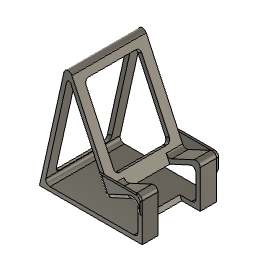
MultimeterStand (Autodesk Fusion 360 design; units mm, degrees)
Autodesk Fusion 360 part; units mm, degrees
sketch "Sketch11" plane through (0, 0, 0) normal (0, 1, 0) x (1, 0, 0)
  line L0 (0, 0) -> (0, -35) construction
  line L1 (0, -35) -> (38.064927, -52.749967)
  line L2 (0, -35) -> (42, -35) construction
  line L3 (38.064927, -52.749967) -> (38.064927, 0)
  line L4 (0, -35) -> (-48.072827, -138.092511)
  line L5 (0, -35) -> (131.25, -35) construction
  line L6 (-48.072827, -138.092511) -> (-53.072827, -138.092511)
  line L7 (0, 0) -> (61.000001, 0) construction
  line L8 (-53.072827, -138.092511) -> (-83.6872, 0)
  line L9 (-53.072827, -138.092511) -> (72.884225, -138.092511) construction
  line L10 (0, 0) -> (-120, 0) construction
  line L11 (-83.6872, 0) -> (38.064927, 0)
  dimension "d68" = 35
  dimension "d69" = 42
  dimension "d70" = 25
  dimension "d71" = 115
  dimension "d72" = 113.75
  dimension "d73" = 5
  dimension "d81" = 102.5
  constraint vertical L0
  constraint coincident L0.start L7.start
  constraint horizontal L2
  constraint vertical L3
  constraint horizontal L5
  constraint horizontal L6
  constraint perpendicular L0 L7
  constraint horizontal L9
  constraint horizontal L10
  constraint coincident L8.end L10
  measures "d68" distance of L0.start L0.end
  measures "d70" angle of L1 L2
  measures "d71" angle of L4 L5
  measures "d81" angle of L8 L9
extrude "Extrude16" add sketch "Sketch11" along normal blind 88 contours L1 L3 L4 L6 L8 L11 picked at (-45.586676, -57.697504) makes body 1
sketch "Sketch12" plane through (38.064927, 0, 0) normal (1, 0, 0) x (0, 1, 0)
  line L0 (0, 52.749967) -> (0, 0)
  line L1 (88, 0) -> (88, 52.749967)
  line L2 (88, 52.749967) -> (0, 52.749967)
  line L3 (44, 52.749967) -> (43.238153, 0) construction
  line L4 (68.619076, 52.749967) -> (18.619076, 52.749967)
  line L5 (18.619076, 52.749967) -> (18.619076, 0)
  line L6 (18.619076, 0) -> (68.619076, 0)
  line L7 (68.619076, 0) -> (68.619076, 52.749967)
  line L8 (68.619076, 52.749967) -> (18.619076, 0) construction
  line L9 (18.619076, 52.749967) -> (68.619076, 0) construction
  line L10 (0, 0) -> (88, 0)
  point P0 (43.619076, 26.374983)
  dimension "d77" = 50
  constraint horizontal L4
  constraint perpendicular L4 L5
  constraint parallel L4 L6
  constraint parallel L5 L7
  constraint collinear L2 L4
extrude "Extrude17" cut sketch "Sketch12" along normal up to surface contours L2 L4 L5 L6 L7 L10 picked at (51.95241, 17.583322) end surface through (0, 0, 35) normal (0.90630779, 0, 0.42261826) offset 0 bodies 1
sketch "Sketch13" plane through (0, 0, 0) normal (0, -1, 0) x (1, 0, 0)
  line L0 (38.064927, 52.749967) -> (0, 35)
  line L1 (0, 35) -> (-48.072827, 138.092511)
  line L2 (-48.072827, 138.092511) -> (-53.072827, 138.092511)
  line L3 (-53.072827, 138.092511) -> (-83.6872, 0)
  line L4 (-83.6872, 0) -> (38.064927, 0)
  line L5 (38.064927, 0) -> (38.064927, 52.749967)
  line L6 (33.064927, 5) -> (33.064927, 44.901539)
  line L7 (33.064927, 44.901539) -> (-2.418448, 28.35537)
  line L8 (-2.418448, 28.35537) -> (-49.768252, 129.897354)
  line L9 (-49.768252, 129.897354) -> (-77.457329, 5)
  line L10 (-77.457329, 5) -> (33.064927, 5)
extrude "Extrude18" cut sketch "Sketch13" against normal up to surface (88 mm away) contours L6 L7 L8 L9 L10 picked at (-43.214676, 54.417574) bodies 1
sketch "Sketch14" plane through (13.405778, 0, 6.251217) normal (0.906308, 0, 0.422618) x (0, 1, 0)
  line L0 (18.619076, 30.468461) -> (68.619076, 30.468461) construction
  line L1 (68.619076, 30.468461) -> (68.619076, 35) construction
  line L2 (68.619076, 35) -> (88, 35) construction
  line L3 (88, 35) -> (88, 138.092511) construction
  line L4 (88, 138.092511) -> (0, 138.092511) construction
  line L5 (0, 138.092511) -> (0, 35) construction
  line L6 (0, 35) -> (18.619076, 35) construction
  line L7 (18.619076, 35) -> (18.619076, 30.468461) construction
  line L8 (0, 138.092511) -> (88, 35) construction
  line L9 (72, 130.296255) -> (16, 130.296255)
  line L10 (11, 125.296255) -> (11, 47.796255)
  line L11 (16, 42.796255) -> (72, 42.796255)
  line L12 (77, 47.796255) -> (77, 125.296255)
  line L13 (77, 130.296255) -> (11, 42.796255) construction
  line L14 (11, 130.296255) -> (77, 42.796255) construction
  line L15 (18.619076, 26.720773) -> (68.619076, 26.720773)
  line L16 (68.619076, 26.720773) -> (68.619076, 31.720773)
  line L17 (68.619076, 31.720773) -> (88, 31.720773)
  line L18 (88, 31.720773) -> (88, 145.470773)
  line L19 (88, 145.470773) -> (0, 145.470773)
  line L20 (0, 145.470773) -> (0, 31.720773)
  line L21 (0, 31.720773) -> (18.619076, 31.720773)
  line L22 (18.619076, 31.720773) -> (18.619076, 26.720773)
  arc A0 (16, 130.296255) -> (11, 125.296255) centre (16, 125.296255) ccw
  arc A1 (77, 125.296255) -> (72, 130.296255) centre (72, 125.296255) ccw
  arc A2 (72, 42.796255) -> (77, 47.796255) centre (72, 47.796255) ccw
  arc A3 (11, 47.796255) -> (16, 42.796255) centre (16, 47.796255) ccw
  point P0 (44, 86.546255)
  dimension "d101" = 66
  dimension "d102" = 87.5
  dimension "d105" = 5
  constraint coincident L2.end L3.start
  constraint horizontal L9
  constraint perpendicular L9 L10
  constraint parallel L9 L11
  constraint parallel L10 L12
  constraint tangent L10 A0
  constraint tangent L9 A0
  constraint tangent L9 A1
  constraint tangent L12 A1
  constraint equal A0 A1
  constraint tangent L12 A2
  constraint tangent L11 A2
  constraint equal A0 A2
  constraint tangent L11 A3
  constraint tangent L10 A3
  constraint equal A0 A3
  measures "d105" radius of A0
fillet "Fillet5" radius 5 6 edges at (38.064927, 78.309538, 52.749967) (38.064927, 9.309538, 52.749967) (0, 9.309538, 35) (0, 78.309538, 35) (-48.072827, 44, 138.092511) (-53.072827, 44, 138.092511) on bodies 1
fillet "Fillet6" radius 2.5 1 edges at (-49.768252, 44, 129.897354) on bodies 1
fillet "Fillet6" radius 5 6 edges at (-77.457329, 44, 5) (33.064927, 9.309538, 5) (33.064927, 78.309538, 5) (33.064927, 78.309538, 44.901539) (33.064927, 9.309538, 44.901539) (-2.418448, 44, 28.35537) on bodies 1
extrude "Extrude19" cut sketch "Sketch14" along normal up to surface contours L9 L10 L11 L12 A0 A1 A2 A3 picked at (33, 99.462922) end surface through (-53.072827, 0, 138.092511) normal (-0.97629601, 0, 0.21643961) offset 0 bodies 1
sketch "Sketch15" plane through (0, 0, 0) normal (0, -1, 0) x (1, 0, 0)
  arc A0 (-4.531539, 32.886909) -> (2.113091, 30.468461) centre (0, 35) ccw
  line L0 (2.113091, 30.468461) -> (25.951836, 41.58465)
  arc A1 (33.064927, 37.053111) -> (25.951836, 41.58465) centre (28.064927, 37.053111) ccw
  line L1 (33.064927, 37.053111) -> (33.064927, 10)
  arc A2 (28.064927, 5) -> (33.064927, 10) centre (28.064927, 10) ccw
  line L2 (28.064927, 5) -> (-71.227458, 5)
  arc A3 (-76.108938, 11.082198) -> (-71.227458, 5) centre (-71.227458, 10) ccw
  line L3 (-76.108938, 11.082198) -> (-51.362279, 122.707165)
  arc A4 (-46.655769, 123.222612) -> (-51.362279, 122.707165) centre (-48.921539, 122.166066) ccw
  line L4 (-46.655769, 123.222612) -> (-4.531539, 32.886909)
  arc A5 (-45.236713, 132.010445) -> (-54.649732, 130.979552) centre (-49.768252, 129.897354) ccw
  line L5 (-54.649732, 130.979552) -> (-83.6872, 0)
  line L6 (-83.6872, 0) -> (38.064927, 0)
  line L7 (38.064927, 0) -> (38.064927, 44.901539)
  arc A6 (38.064927, 44.901539) -> (30.951836, 49.433078) centre (33.064927, 44.901539) ccw
  line L8 (30.951836, 49.433078) -> (4.531539, 37.113091)
  arc A7 (-2.113091, 39.531539) -> (4.531539, 37.113091) centre (2.418448, 41.64463) ccw
  line L9 (-2.113091, 39.531539) -> (-45.236713, 132.010445)
  line L10 (38.064927, 30) -> (-9.500954, 30) construction
  line L11 (38.064927, 30) -> (-12.465591, 30)
  line L12 (-12.465591, 30) -> (-12.465591, 49.901539)
  line L13 (-12.465591, 49.901539) -> (38.064927, 49.901539)
  line L14 (38.064927, 49.901539) -> (38.064927, 30)
  constraint horizontal L10
  constraint tangent A0 L10
  constraint horizontal L11
  constraint vertical L12
  constraint horizontal L13
  constraint vertical L14
  constraint tangent A6 L13
ref_plane "WorkPlane4" through (-22.811136, 44, 67.62885) normal (0, -1, 0) x (-1, 0, 0)
extrude "Extrude20" add sketch "Sketch15" along normal blind 2.5 separate body contours A0 L0 A1 L1 L4 L7 A6 L8 A7 L9 L11 L13 L14 | A6 L8 A7 L9 L13 picked at (20.478403, 42.710273) picked at (9.511558, 45.482569) makes body 2
fillet "Fillet7" radius 5 6 edges at (-8.498565, -2.5, 41.394224) (-1.710101, -2.5, 30.301537) (14.032464, -2.5, 36.026556) (30.751425, -2.5, 41.270068) (33.064927, -2.5, 33.526556) (35.564927, -2.5, 30) on bodies 2
mirror "Mirror5" about plane through (-22.811136, 44, 67.62885) normal (0, -1, 0) of bodies 2 makes body 3
equation "DeviceWidth = 88 mm"
equation "DeviceBottomThickness = 42 mm"
equation "Angle = 25 deg"
equation "DeviceHeight = 175 mm"
equation "WallThickness = 5 mm"
equation "ProbeDiameter = 9.7 mm"
equation "d69 = DeviceBottomThickness"
equation "d70 = Angle"
equation "d71 = Angle + 90 deg"
equation "d72 = DeviceHeight * 0.65"
equation "d73 = WallThickness"
equation "d74 = DeviceWidth"
equation "d81 = 90 deg + Angle / 2"
equation "d82 = -WallThickness"
equation "d86 = WallThickness"
equation "d96 = WallThickness"
equation "d100 = WallThickness / 2"
equation "d101 = DeviceWidth * 0.75"
equation "d102 = DeviceHeight * 0.5"
equation "d105 = WallThickness"
equation "d106 = WallThickness * 0.5"
equation "d109 = WallThickness"
named bodies: "MultimeterHolder", "LeftLimiter", "RightLimiter"
